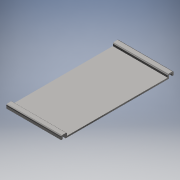
# Autodesk Inventor part: Gondola Base Plate
Saved by Autodesk Inventor 2018 (Build 220112000, 112)
## iProperties
Created: 2018-02-09
Part Number: Gondola Base Plate
Material: Steel, Alloy
Document SubType Name: Modeling
Designer: Joey
Density: 7.73 g/cm^3
Appearance: Diamond Plate
Author: Joey
Autodesk Inventor part; units mm, degrees
ref_plane "YZ Plane" through (0, 0, 0) normal (1, 0, 0) x (0, 1, 0)
ref_plane "XZ Plane" through (0, 0, 0) normal (0, 1, 0) x (-1, 0, 0)
ref_plane "XY Plane" through (0, 0, 0) normal (0, 0, 1) x (1, 0, 0)
sketch "Sketch1" plane through (0, 0, 0) normal (1, 0, 0) x (0, 1, 0)
  line L0 (-12.7, 939.8) -> (-12.7, 914.4)
  line L1 (-12.7, 914.4) -> (25.4, 914.4)
  line L2 (25.4, 914.4) -> (25.4, 863.6)
  line L3 (25.4, -914.4) -> (-12.7, -914.4)
  line L4 (-12.7, -914.4) -> (-12.7, -939.8)
  line L5 (-12.7, -939.8) -> (50.8, -939.8)
  line L6 (50.8, -939.8) -> (50.8, -838.2)
  line L7 (50.8, 939.8) -> (-12.7, 939.8)
  line L8 (25.4, 863.6) -> (-25.4, 863.6)
  line L9 (-25.4, 863.6) -> (-25.4, -863.6)
  line L10 (-25.4, -863.6) -> (25.4, -863.6)
  line L11 (25.4, -863.6) -> (25.4, -914.4)
  line L12 (25.4, 863.6) -> (25.4, -863.6) construction
  line L13 (50.8, -838.2) -> (0, -838.2)
  line L14 (0, -838.2) -> (0, 838.2)
  line L15 (0, 838.2) -> (50.8, 838.2)
  line L16 (50.8, 838.2) -> (50.8, 939.8)
  line L17 (50.8, -838.2) -> (50.8, 838.2) construction
  point P0 (0, 0)
  point P1 (0, 0)
  point P2 (0, 0)
  dimension "d4" = 25.4
  dimension "d5" = 1879.6
  dimension "d7" = 63.5
  dimension "d11" = 50.8
  dimension "d12" = 50.8
  dimension "d13" = 50.8
  dimension "d14" = 76.2
  dimension "d15" = 25.4
  dimension "d16" = 25.4
  dimension "d17" = 25.4
  constraints: 36 end point, 19 perpendicular, 2 coincident, 2 horizontal, 2 point on line, 1 collinear, 1 midpoint, 1 parallel, 1 vertical
  measures "d4" distance of L3.end L4.end
  measures "d5" distance of L5.end L7.start
  measures "d7" distance between parallel lines of L4 L6
  measures "d11" distance between parallel lines of L8 L1
  measures "d12" distance between parallel lines of L10 L3
  measures "d13" distance of L9.end L10.end
  measures "d14" distance between parallel lines of L9 L6
  measures "d15" distance between parallel lines of L13 L10
  measures "d16" distance between parallel lines of L9 L14
  measures "d17" distance between parallel lines of L15 L8
extrude "Extrusion1" add sketch "Sketch1" along normal mid plane 914.4
fillet "Fillet1" radius 25.4 4 edges at (0, 50.8, 939.8) (0, 50.8, -939.8) (0, 50.8, -838.2) (0, 50.8, 838.2)
body "Solid1"
